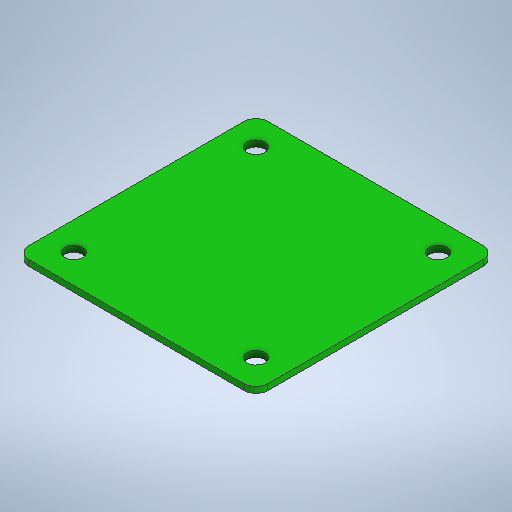
# Autodesk Inventor part: CHIP
Saved by Autodesk Inventor 2025.2 (Build 292293000, 293)
## iProperties
Created: 2025-05-07
Part Number: CHIP
Material: Generic
Document SubType Name: Modeling
Designer: joaki
Density: 1 g/cm^3
Appearance: Default
Author: joaki
Autodesk Inventor part; units mm, degrees
ref_plane "YZ Plane" through (0, 0, 0) normal (1, 0, 0) x (0, 1, 0)
ref_plane "XZ Plane" through (0, 0, 0) normal (0, 1, 0) x (-1, 0, 0)
ref_plane "XY Plane" through (0, 0, 0) normal (0, 0, 1) x (1, 0, 0)
sketch "Sketch1" plane through (0, 0, 0) normal (0, 1, 0) x (-1, 0, 0)
  line L0 (14.9302, 26.8372) -> (-25.0698, 26.8372)
  line L1 (-25.0698, 26.8372) -> (-25.0698, -13.1628)
  line L2 (-25.0698, -13.1628) -> (14.9302, -13.1628)
  line L3 (14.9302, -13.1628) -> (14.9302, 26.8372)
  line L4 (-5.0698, 26.8372) -> (-5.0698, -13.1628)
  line L5 (14.9302, 6.8372) -> (-25.0698, 6.8372)
  circle A0 centre (10.1802, -8.4128) radius 1.5
  circle A1 centre (10.1802, 22.0872) radius 1.5
  circle A2 centre (-20.3198, 22.0872) radius 1.5
  circle A3 centre (-20.3198, -8.4128) radius 1.5
  point P0 (0, 0)
  dimension "d0" = 40
  dimension "d1" = 40
  dimension "d2" = 3
  dimension "d3" = 3
  dimension "d4" = 3
  dimension "d5" = 3
  dimension "d6" = 30.5
  dimension "d7" = 30.5
  dimension "d8" = 30.5
  dimension "d9" = 30.5
  dimension "d10" = 15.25
  dimension "d11" = 15.25
  dimension "d12" = 15.25
  dimension "d13" = 15.25
  constraints: 12 end point, 4 centre point, 4 midpoint, 2 parallel, 1 horizontal, 1 perpendicular
  measures "d0" distance of L2.end L0.start
  measures "d1" distance of L1.end L2.end
  measures "d2" diameter of A0
  measures "d3" diameter of A1
  measures "d4" diameter of A2
  measures "d5" diameter of A3
  measures "d6" distance of A0.centre A3.centre
  measures "d7" distance of A2.centre A1.centre
  measures "d8" distance of A0.centre A1.centre
  measures "d9" distance of A3.centre A2.centre
  measures "d10" distance from line of L4 A0.centre
  measures "d11" distance from line of L5 A0.centre
  measures "d12" distance from line of L4 A1.centre
  measures "d13" distance from line of L5 A2.centre
extrude "Extrusion1" add sketch "Sketch1" along normal blind 1
fillet "Fillet1" radius 2 4 edges at (-14.9302, 0.5, 26.8372) (25.0698, 0.5, 26.8372) (25.0698, 0.5, -13.1628) (-14.9302, 0.5, -13.1628)
body "Solid1"
